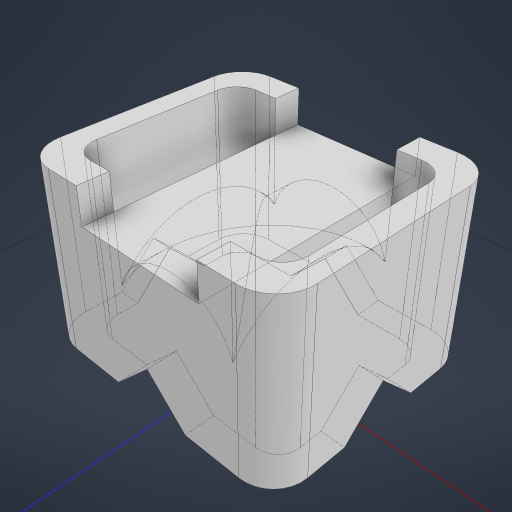
# Autodesk Inventor part: Richtfest
Saved by Autodesk Inventor 2023 (Build 270158030, 158C)
## iProperties
Created: 2022-05-12
Part Number: Richtfest
Material: Generic
Document SubType Name: Modeling
Designer: Simon
Density: 1 g/cm^3
Appearance: Default
Author: Simon
Autodesk Inventor part; units mm, degrees
ref_plane "YZ Plane" through (0, 0, 0) normal (1, 0, 0) x (0, 1, 0)
ref_plane "XZ Plane" through (0, 0, 0) normal (0, 1, 0) x (-1, 0, 0)
ref_plane "XY Plane" through (0, 0, 0) normal (0, 0, 1) x (1, 0, 0)
sketch "Sketch1" plane through (0, 0, 0) normal (0, 1, 0) x (-1, 0, 0)
  line L0 (5.5, 10) -> (-5.5, 10)
  line L1 (-5.5, 10) -> (-5.5, -10)
  line L2 (-5.5, -10) -> (5.5, -10)
  line L3 (5.5, -10) -> (5.5, 10)
  line L4 (5.5, 10) -> (-5.5, -10) construction
  line L5 (-5.5, 10) -> (5.5, -10) construction
  point P0 (0, 0)
  dimension "d0" = 11
  dimension "d1" = 20
  constraints: 12 end point, 2 midpoint, 2 parallel, 1 horizontal, 1 perpendicular
  measures "d0" distance of L2.end L1.end
  measures "d1" distance of L1.end L0.end
extrude "Extrusion1" add sketch "Sketch1" along normal mid plane 2
sketch "Sketch2" plane through (0, -1, 0) normal (0, -1, 0) x (1, 0, 0)
  line L0 (5.5, -10) -> (5.5, 10) projected
  line L1 (5.5, 10) -> (-5.5, 10) projected
  line L2 (-5.5, 10) -> (-5.5, -10) projected
  line L3 (-5.5, -10) -> (5.5, -10) projected
  line L4 (-5.5, 5.5) -> (5.5, 5.5)
  line L5 (5.5, 5.5) -> (5.5, -5.5)
  line L6 (5.5, -5.5) -> (-5.5, -5.5)
  line L7 (-5.5, -5.5) -> (-5.5, 5.5)
  line L8 (-5.5, 5.5) -> (5.5, -5.5) construction
  line L9 (5.5, 5.5) -> (-5.5, -5.5) construction
  point P0 (0, 0)
  dimension "d4" = 11
  dimension "d5" = 11
  constraints: 12 end point, 2 midpoint, 2 parallel, 1 horizontal, 1 perpendicular
  measures "d4" distance of L5.end L6.end
  measures "d5" distance of L4.end L5.end
extrude "Extrusion2" add sketch "Sketch2" along normal blind 10 contours L3 L2 L6 L0 | L4 L2 L1 L0
sketch "Sketch3" plane through (0, 1, 0) normal (0, 1, 0) x (1, 0, 0)
  line L0 (-5.5, 5.5) -> (5.5, 5.5) projected
  line L1 (5.5, -5.5) -> (-5.5, -5.5) projected
  line L2 (-5.5, -10) -> (5.5, -10) projected
  line L3 (5.5, -10) -> (9.5, -10)
  line L4 (9.5, -10) -> (9.5, 10)
  line L5 (9.5, 10) -> (5.5, 10)
  line L6 (5.5, 10) -> (5.5, -10)
  line L7 (5.5, -5.5) -> (9.5, -5.5)
  line L8 (9.5, -5.5) -> (9.5, 5.5)
  line L9 (9.5, 5.5) -> (5.5, 5.5)
  line L10 (5.5, 5.5) -> (5.5, -5.5)
  line L11 (9.5, -10) -> (11.5, -10)
  line L12 (11.5, -10) -> (11.5, 10)
  line L13 (11.5, 10) -> (9.5, 10)
  line L14 (9.5, 10) -> (9.5, -10)
  point P0 (0, 0)
  dimension "d8" = 4
  dimension "d9" = 20
  dimension "d10" = 2
  dimension "d11" = 20
  constraints: 24 end point, 6 parallel, 3 horizontal, 3 perpendicular, 1 point on line
  measures "d8" distance of L5.end L4.end
  measures "d9" distance of L4.end L3.end
  measures "d10" distance of L13.end L12.end
  measures "d11" distance of L12.end L11.end
extrude "Extrusion3" add sketch "Sketch3" along normal blind 3 and the other way blind 12 contours L6 L7 L4 L3 | L4 L13 L12 L11 | L6 L5 L4 L9
move faces "Move1" translate (0, 0, -2) faces at (3.1667, -7.6667, -5.5)
move faces "Move2" translate (0, 0, 2) faces at (3.1667, -7.6667, 5.5)
mirror "Mirror1" about plane through (0, 0, 0) normal (1, 0, 0)
sketch "Sketch4" plane through (5.5, 4, 10) normal (0, 0, 1) x (1, 0, 0)
  line L0 (-8, -17) -> (-3, -17)
  line L1 (-3, -17) -> (-3, -13)
  line L2 (-3, -13) -> (-8, -13)
  line L3 (-8, -13) -> (-8, -17)
  line L4 (4, -15) -> (-15, -15) projected
  line L5 (-8, -17) -> (-3, -13) construction
  line L6 (-3, -17) -> (-8, -13) construction
  point P0 (-5.5, -4)
  point P1 (-5.5, -15)
  point P2 (-8, -15)
  point P3 (-3, -15)
  dimension "d22" = 5
  dimension "d23" = 4
  constraints: 12 end point, 3 midpoint, 2 parallel, 1 horizontal, 1 perpendicular
  measures "d22" distance of L2.end L1.end
  measures "d23" distance of L1.end L0.end
extrude "Extrusion4" cut sketch "Sketch4" along normal mid plane 9 contours L3 L2 L1 L4
pattern_circular "Circular Pattern1" count 4 over 360 about axis through (0, -10, 0) along (0, 1, 0) of "Extrusion4"
sketch "Sketch5" plane through (-5.5, -1, -7.5) normal (0, 0, 1) x (1, 0, 0)
  line L0 (0, 0) -> (11, 0) projected
  line L1 (11, 0) -> (0, 0)
  line L2 (0, 0) -> (0, -4)
  line L3 (0, -4) -> (11, -4)
  line L4 (11, -4) -> (11, 0)
  arc A0 (11, -4) -> (0, -4) centre (5.5, -5.7812) ccw
  point P0 (5.5, 1)
  point P1 (5.5, 0)
  dimension "d29" = 11
  dimension "d30" = 4
  constraints: 8 end point, 2 parallel, 2 point on circle, 1 centre point, 1 horizontal, 1 perpendicular
  measures "d29" distance of L3.end L2.end
  measures "d30" distance of L2.end L1.end
extrude "Extrusion5" add sketch "Sketch5" along normal up to surface (15 mm away) contours L0 A0 L2 | L0 L4 A0
sketch "Sketch6" plane through (-5.5, 1, -7.5) normal (-1, 0, 0) x (0, 0, 1)
  line L0 (15, -6) -> (15, 0) projected
  line L1 (0, -6) -> (15, -6) projected
  arc A0 (15, -6) -> (0, -6) centre (7.5, -11.0312) ccw
  line L2 (15, -2) -> (0, -2) projected
  line L3 (0, -12) -> (0, 3) projected
  line L4 (15, -12) -> (15, 3) projected
  line L5 (15, -2) -> (0, -2) projected
  point P0 (7.5, -1)
  constraints: 2 point on circle, 1 centre point
extrude "Extrusion6" cut sketch "Sketch6" against normal blind 11 contours L1 A0
fillet "Fillet1" radius 2 4 edges at (-9.5, -3.5, 7.5) (-9.5, -3.5, -7.5) (9.5, -3.5, -7.5) (9.5, -3.5, 7.5)
chamfer "Chamfer1" distance 1 angle 45 16 edges at (2.5, -9, -8.75) (2.5, -11, -8.75) (-2.5, -11, -8.75) (-2.5, -9, -8.75) (-10.5, -9, -2.5) (-10.5, -11, -2.5) (-10.5, -11, 2.5) (-10.5, -9, 2.5) (-2.5, -9, 8.75) (-2.5, -11, 8.75) (2.5, -9, 8.75) (2.5, -11, 8.75) (10.5, -9, 2.5) (10.5, -11, 2.5) (10.5, -9, -2.5) (10.5, -11, -2.5)
delete faces "Delete Face1" heal yes whole lump no faces at (0.5, -9, 8.3333) (-10.1667, -9, 0.5) (-0.5, -9, -8.3333) (10.8333, -9, -0.5)
fillet "Fillet2" radius 3 4 edges at (11.5, -3.5, 10) (-11.5, -3.5, 10) (-11.5, -3.5, -10) (11.5, -3.5, -10)
body "Solid1"
